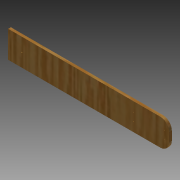
# Autodesk Inventor part: segment1b
Saved by Autodesk Inventor 2013 (Build 170138000, 138)
## iProperties
Created: 2014-10-10
Part Number: segment1b
Material: Plywood, Finish
Document SubType Name: Modeling
Designer: Masta
Density: 0.552 g/cm^3
Mass: 56.9255 g
Surface Area: 405.946 cm^2
Volume: 103.126 cm^3
Author: Masta
Autodesk Inventor part; units mm, degrees
ref_plane "YZ Plane" through (0, 0, 0) normal (1, 0, 0) x (0, 1, 0)
ref_plane "XZ Plane" through (0, 0, 0) normal (0, 1, 0) x (-1, 0, 0)
ref_plane "XY Plane" through (0, 0, 0) normal (0, 0, 1) x (1, 0, 0)
sketch "Sketch1" plane through (0, 0, 0) normal (0, 1, 0) x (-1, 0, 0)
  line L0 (0, 0) -> (-16.25, 0)
  line L1 (0, 0) -> (46.75, 0)
  line L2 (300, 0) -> (330, 0)
  line L3 (330, 30) -> (-30, 30)
  line L4 (-19.25, 8.5) -> (49.75, 8.5) construction
  line L5 (49.75, 8.5) -> (49.75, -8.5) construction
  line L6 (49.75, -8.5) -> (-19.25, -8.5) construction
  line L7 (-19.25, -8.5) -> (-19.25, 8.5) construction
  line L8 (-19.25, 8.5) -> (49.75, -8.5) construction
  line L9 (49.75, 8.5) -> (-19.25, -8.5) construction
  line L10 (-30, 0) -> (-30, 30)
  line L11 (330, 0) -> (330, 30)
  line L12 (46.75, 0) -> (300, 0)
  line L13 (-16.25, 0) -> (-30, 0)
  line L14 (0, 0) -> (-30, 0) construction
  point P0 (15.25, 0)
  point P1 (15.25, 0)
  dimension "d0" = 300
  dimension "d7" = 69
  dimension "d8" = 17
  dimension "d10" = 30
  dimension "d11" = 30
  dimension "d29" = 19.25
  constraints: 30 end point, 5 collinear, 4 coincident, 4 parallel, 3 horizontal, 3 perpendicular, 2 midpoint, 2 point on line
  measures "d0" distance of L0.start L2.start
  measures "d7" distance of L5.end L6.end
  measures "d8" distance of L4.end L5.end
  measures "d10" distance of L10.start L3.end
  measures "d11" distance of L2.end L3.start
  measures "d29" distance from line of point (0, 0) L7
extrude "Extrusion1" add sketch "Sketch1" along normal blind 6
hole "Hole1" at (19.25, 0, 8.5) at (-49.75, 0, 8.5) direction (0, 1, 0) diameter 2 end through all
hole "Hole2" at (-300, 0, 0) direction (0, 1, 0) diameter 3 end through all
fillet "Fillet1" radius 20 1 edges at (30, 3, 30)
mirror "Mirror1" about plane through (16.25, 0, 0) normal (0, 0, -1)
body "Solid1"
